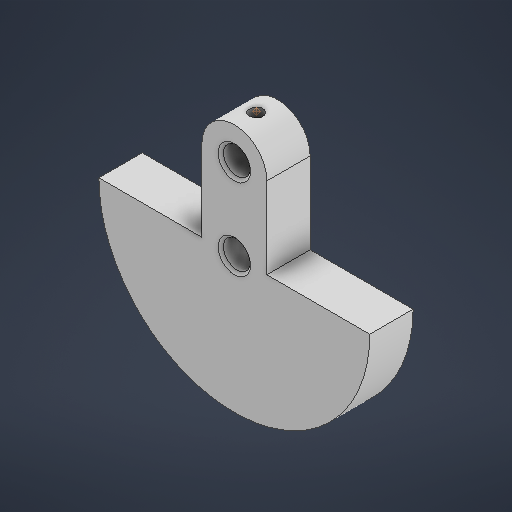
# Autodesk Inventor part: Counterweight
Saved by Autodesk Inventor 2025.4 (Build 294407000, 407)
## iProperties
Created: 2026-05-29
Part Number: Counterweight
Material: Generic
Document SubType Name: Modeling
Designer: VuQuan
Density: 1 g/cm^3
Appearance: Default
Author: VuQuan
Autodesk Inventor part; units mm, degrees
note: some values were not read from the file. Chosen so that the rebuilt part matches the saved one: direction of "Hole1".
ref_plane "YZ Plane" through (0, 0, 0) normal (1, 0, 0) x (0, 1, 0)
ref_plane "XZ Plane" through (0, 0, 0) normal (0, 1, 0) x (-1, 0, 0)
ref_plane "XY Plane" through (0, 0, 0) normal (0, 0, 1) x (1, 0, 0)
sketch "Sketch1" plane through (0, 0, 0) normal (0, 0, 1) x (1, 0, 0)
  arc A0 (-25, 0) -> (25, 0) centre (0, 0) ccw
  circle A1 centre (0, 0) radius 2.5
  circle A2 centre (0, 15) radius 2.5
  line L0 (-25, 0) -> (-6, 0)
  line L1 (-6, 0) -> (-6, 15)
  arc A3 (6, 15) -> (-6, 15) centre (0, 15) ccw
  line L2 (6, 15) -> (6, 0)
  line L3 (6, 0) -> (25, 0)
  point P0 (0, 21)
  dimension "d0" = 50
  dimension "d1" = 5
  dimension "d2" = 15
  dimension "d4" = 12
  constraints: 8 end point, 5 point on circle, 4 centre point, 3 coincident, 3 point on line, 2 tangent, 1 equal radius, 1 horizontal, 1 parallel, 1 perpendicular, 1 vertical alignment
  measures "d0" diameter of A0
  measures "d1" diameter of A1
  measures "d2" distance of point (0, 0) A2.centre
  measures "d4" distance between parallel lines of L1 L2
extrude "Extrusion1" add sketch "Sketch1" along normal mid plane 8
hole "Hole1" at (0, 21, 0) direction (0, -1, 0) diameter 2.459 end up to surface thread size "M3x0.5" class "6H" standard "ISO Metric profile"
chamfer "Chamfer1" distance 0.5 angle 45 4 edges at (-2.5, 15, 4) (-2.5, 0, 4) (-2.5, 0, -4) (-2.5, 15, -4)
body "Solid1"
